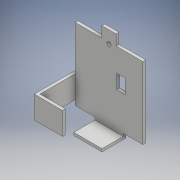
# Autodesk Inventor part: arm_2_case
Saved by Autodesk Inventor 2018 (Build 220112000, 112)
## iProperties
Created: 2018-02-08
Part Number: arm_2_case
Material: Genérico
Document SubType Name: Modeling
Designer: se_ma
Density: 1 g/cm^3
Appearance: Valor por defecto
Author: se_ma
Autodesk Inventor part; units mm, degrees
ref_plane "YZ Plane" through (0, 0, 0) normal (1, 0, 0) x (0, 1, 0)
ref_plane "XZ Plane" through (0, 0, 0) normal (0, 1, 0) x (-1, 0, 0)
ref_plane "XY Plane" through (0, 0, 0) normal (0, 0, 1) x (1, 0, 0)
sketch "Boceto1" plane through (0, 0, 0) normal (0, 1, 0) x (-1, 0, 0)
  line L0 (48, 0) -> (48, -51)
  line L1 (48, -51) -> (0, -51)
  line L2 (0, -51) -> (0, 0)
  line L3 (24, 7.5) -> (29, 7.5)
  line L4 (29, 7.5) -> (29, 0)
  line L5 (24, 7.5) -> (19, 7.5)
  line L6 (19, 7.5) -> (19, 0)
  line L7 (24, 7.5) -> (24, -1.25)
  circle A0 centre (24, -1.25) radius 1.5
  line L8 (29, 0) -> (48, 0)
  line L9 (19, 0) -> (0, 0)
  dimension "d0" = 48
  dimension "d1" = 51
  dimension "d3" = 5
  dimension "d4" = 5
  dimension "d5" = 8.75
  dimension "d6" = 3
  constraints: 20 end point, 2 equal length, 1 centre point, 1 coincident, 1 horizontal, 1 point on line, 1 vertical
  measures "d0" distance of L0.end L1.end
  measures "d1" distance of L0.start L0.end
  measures "d3" distance of L3.start L3.end
  measures "d4" distance of L3.start L5.end
  measures "d5" distance of L3.start L7.end
  measures "d6" diameter of A0
extrude "Extrusión1" add sketch "Boceto1" along normal blind 2
sketch "Boceto2" plane through (-48, 0, -51) normal (-1, 0, 0) x (0, 0, 1)
  line L0 (51, 0) -> (0, 0) projected
  line L1 (0, 0) -> (3.5, 0)
  line L2 (3.5, 0) -> (3.5, -25)
  line L3 (3.5, 0) -> (28.5, 0) construction
  line L4 (3.5, -25) -> (19.5, -25)
  line L5 (19.5, -25) -> (19.5, 0)
  line L6 (19.5, 0) -> (3.5, 0)
  line L7 (19.5, 0) -> (19.5, 2)
  line L8 (51, 2) -> (0, 2) projected
  line L9 (19.5, 2) -> (3.5, 2)
  line L10 (3.5, 2) -> (3.5, 0)
  dimension "d9" = 3.5
  dimension "d10" = 25
  dimension "d11" = 90
  dimension "d12" = 16
  constraints: 18 end point, 4 perpendicular, 4 point on line, 2 horizontal, 2 vertical
  measures "d9" distance of L0.end L1.end
  measures "d10" distance of L1.end L2.end
  measures "d11" angle of L2 L3
  measures "d12" distance of L2.end L4.end
extrude "Extrusión2" add sketch "Boceto2" along normal blind 2
sketch "Boceto3" plane through (-48, -25, -47.5) normal (0, -1, 0) x (1, 0, 0)
  line L0 (-2, 0) -> (-2, 16) projected
  line L1 (-2, 0) -> (18, 0)
  line L2 (18, 0) -> (18, 16)
  line L3 (0, 16) -> (-2, 16) projected
  line L4 (18, 16) -> (-2, 16)
  point P0 (48, 47.5)
  dimension "d15" = 20
  constraints: 6 end point, 2 perpendicular, 1 horizontal
  measures "d15" distance of L0.start L1.end
extrude "Extrusión3" add sketch "Boceto3" along normal blind 2
sketch "Boceto4" plane through (0, 2, 0) normal (0, 1, 0) x (1, 0, 0)
  line L0 (0, 51) -> (-48, 51) projected
  line L1 (-24, 51) -> (-24, 53)
  line L2 (-24, 53) -> (-34, 53)
  line L3 (-34, 53) -> (-34, 51)
  line L4 (-34, 51) -> (-14, 51)
  line L5 (-14, 51) -> (-14, 53)
  line L6 (-14, 53) -> (-24, 53)
  point P0 (0, 0)
  dimension "d18" = 2
  dimension "d19" = 10
  dimension "d20" = 20
  constraints: 12 end point, 5 perpendicular, 2 point on line, 1 midpoint, 1 vertical
  measures "d18" distance of L1.start L1.end
  measures "d19" distance of L1.end L2.end
  measures "d20" distance of L3.end L4.end
extrude "Extrusión4" add sketch "Boceto4" against normal blind 2
sketch "Boceto5" plane through (-14, 2, -53) normal (0, 0, -1) x (-1, 0, 0)
  line L0 (0, 0) -> (20, 0) projected
  line L1 (20, 0) -> (20, -17)
  line L2 (20, -17) -> (0, -17)
  line L3 (0, 0) -> (0, -2) projected
  line L4 (0, -17) -> (0, 0)
  line L5 (20, 0) -> (20, -2) projected
  line L6 (0, 0) -> (20, 0)
  point P0 (-14, -2)
  dimension "d23" = 17
  constraints: 8 end point, 2 perpendicular, 1 collinear, 1 vertical
  measures "d23" distance of L0.end L1.end
extrude "Extrusión5" add sketch "Boceto5" along normal blind 2
sketch "Boceto6" plane through (0, 2, 0) normal (0, 1, 0) x (1, 0, 0)
  line L0 (-48, 47.5) -> (-48, 31.5) projected
  line L1 (-48, 47.5) -> (-18.5, 47.5)
  line L2 (-18.5, 47.5) -> (-18.5, 26.5)
  line L3 (-18.5, 26.5) -> (-18.5, 16.5)
  line L4 (-18.5, 16.5) -> (-12.5, 16.5)
  line L5 (-12.5, 16.5) -> (-12.5, 26.5)
  line L6 (-12.5, 26.5) -> (-18.5, 26.5)
  point P0 (0, 0)
  dimension "d26" = 29.5
  dimension "d27" = 21
  dimension "d28" = 10
  dimension "d29" = 6
  constraints: 12 end point, 4 perpendicular, 1 horizontal, 1 vertical
  measures "d26" distance of L0.start L1.end
  measures "d27" distance of L1.end L2.end
  measures "d28" distance of L2.end L3.end
  measures "d29" distance of L3.end L4.end
extrude "Extrusión6" cut sketch "Boceto6" against normal blind 2
